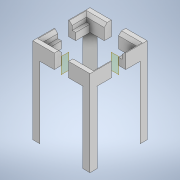
# Autodesk Inventor part: soporte_stm
Saved by Autodesk Inventor 2021 (Build 250183000, 183)
## iProperties
Created: 2022-03-28
Part Number: soporte_stm
Material: Genérico
Document SubType Name: Modeling
Designer: orgyn
Density: 1 g/cm^3
Appearance: Valor por defecto
Author: orgyn
Autodesk Inventor part; units mm, degrees
ref_plane "YZ Plane" through (0, 0, 0) normal (1, 0, 0) x (0, 1, 0)
ref_plane "XZ Plane" through (0, 0, 0) normal (0, 1, 0) x (-1, 0, 0)
ref_plane "XY Plane" through (0, 0, 0) normal (0, 0, 1) x (1, 0, 0)
sketch "Boceto1" plane through (0, 0, 0) normal (0, 1, 0) x (-1, 0, 0)
  line L0 (0, 0) -> (10, 0)
  line L1 (10, 0) -> (10, -5)
  line L2 (10, -5) -> (0, -5)
  line L3 (0, -5) -> (0, -15)
  line L4 (0, -15) -> (-5, -15)
  line L5 (-5, -15) -> (-5, 0)
  line L6 (-5, 0) -> (10, 0)
  line L7 (0, -5) -> (-2.5, -5)
  line L8 (-2.5, -5) -> (-2.5, -15)
  dimension "d0" = 10
  dimension "d1" = 5
  dimension "d2" = 10
  dimension "d3" = 5
  dimension "d4" = 2.5
  constraints: 18 end point, 5 perpendicular, 2 horizontal, 1 collinear, 1 midpoint, 1 point on line
  measures "d0" distance of L0.start L0.end
  measures "d1" distance of L0.end L1.end
  measures "d2" distance of L2.end L3.end
  measures "d3" distance of L3.end L4.end
  measures "d4" distance of L2.end L7.end
extrude "Extrusión1" add sketch "Boceto1" along normal blind 10
sketch "Boceto2" plane through (0, 10, 0) normal (0, 1, 0) x (1, 0, 0)
  line L0 (0, 15) -> (0, 5) projected
  line L1 (0, 5) -> (2.5, 5)
  line L2 (2.5, 5) -> (2.5, 15)
  line L3 (5, 15) -> (0, 15) projected
  point P0 (0, 0)
  dimension "d7" = 2.5
  constraints: 4 end point, 1 horizontal, 1 midpoint
  measures "d7" distance of L0.end L1.end
extrude "Extrusión2" cut sketch "Boceto2" against normal blind 5
sketch "Boceto3" plane through (0, 0, 0) normal (0, -1, 0) x (1, 0, 0)
  line L0 (0, -5) -> (-10, -5) projected
  line L1 (0, -5) -> (5, -5)
  line L2 (5, 0) -> (5, -15) projected
  line L3 (5, 0) -> (5, -5)
  line L4 (5, 0) -> (0, 0)
  line L5 (-10, 0) -> (5, 0) projected
  line L6 (0, -5) -> (0, 0)
  line L7 (5, -5) -> (0, 0)
  constraints: 10 end point, 2 perpendicular, 1 collinear, 1 horizontal, 1 point on line
extrude "Extrusión3" add sketch "Boceto3" along normal blind 50 contours L7 L4 L2
chamfer "Chaflán1" distance 2 angle 45 2 edges at (2.5, 10, -10) (-3.75, 10, -5)
ref_plane "Plano de trabajo1" through (-15, 0, -5) normal (-1, 0, 0) x (0, 0, 1)
ref_plane "Plano de trabajo2" through (5, 0, -20) normal (0, 0, -1) x (-1, 0, 0)
mirror "Simetría1" about plane through (5, 0, -20) normal (0, 0, -1)
mirror "Simetría2" about plane through (-15, 0, -5) normal (-1, 0, 0)
